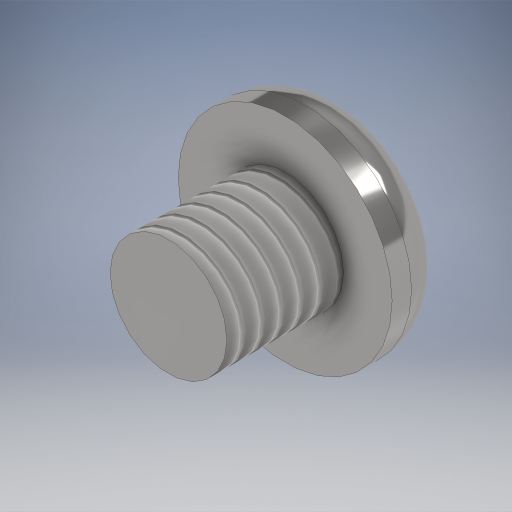
# Autodesk Inventor part: Болт М3 4мм
Saved by Autodesk Inventor 2023 (Build 270158000, 158)
## iProperties
Created: 2022-12-28
Part Number: Болт М3 4мм
Material: Типовые
Document SubType Name: Modeling
Designer: Admin
Density: 1 g/cm^3
Appearance: По умолчанию
Author: Admin
Autodesk Inventor part; units mm, degrees
ref_plane "YZ Plane" through (0, 0, 0) normal (1, 0, 0) x (0, 1, 0)
ref_plane "XZ Plane" through (0, 0, 0) normal (0, 1, 0) x (-1, 0, 0)
ref_plane "XY Plane" through (0, 0, 0) normal (0, 0, 1) x (1, 0, 0)
sketch "Эскиз1" plane through (0, 0, 0) normal (0, 0, 1) x (1, 0, 0)
  circle A0 centre (0, 0) radius 1.5
  circle A1 centre (0, 0) radius 2.75
  dimension "d0" = 5.5
  dimension "d1" = 3
  constraints: 2 centre point, 2 coincident
  measures "d0" diameter of A1
  measures "d1" diameter of A0
extrude "Выдавливание1" add sketch "Эскиз1" along normal blind 3 contours A0
extrude "Выдавливание2" add sketch "Эскиз1" against normal blind 1.5 contours A0 | A1
thread "Резьба1" size "M3x0.5" class "6g" standard "ISO Metric profile" full length
sketch "Эскиз2" plane through (0, 0, -1.5) normal (0, 0, -1) x (-1, 0, 0)
  line L0 (0, 1.1547) -> (1, 0.5774)
  line L1 (1, 0.5774) -> (1, -0.5774)
  line L2 (1, -0.5774) -> (0, -1.1547)
  line L3 (0, -1.1547) -> (-1, -0.5774)
  line L4 (-1, -0.5774) -> (-1, 0.5774)
  line L5 (-1, 0.5774) -> (0, 1.1547)
  point P0 (0, 0)
  point P1 (0, 0)
  dimension "d8" = 2
  constraints: 12 end point, 1 coincident, 1 vertical, 13 other
  measures "d8" distance between parallel lines of L4 L1
extrude "Выдавливание3" cut sketch "Эскиз2" against normal blind 1
fillet "Сопряжение1" radius 1 1 edges at (-2.75, 0, -1.5)
